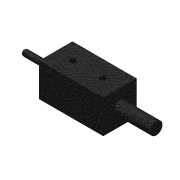
# Autodesk Inventor part: 00_JF-0530B-solenoid
Saved by Autodesk Inventor 2019.4 (Build 234330000, 330)
## iProperties
Created: 2020-11-20
Part Number: 00_JF-0530B-solenoid
Material: Generic
Document SubType Name: Modeling
Designer: diederichbenedict
Density: 1 g/cm^3
Appearance: Black Cast
Author: diederichbenedict
Autodesk Inventor part; units mm, degrees
ref_plane "YZ Plane" through (0, 0, 0) normal (1, 0, 0) x (0, 1, 0)
ref_plane "XZ Plane" through (0, 0, 0) normal (0, 1, 0) x (-1, 0, 0)
ref_plane "XY Plane" through (0, 0, 0) normal (0, 0, 1) x (1, 0, 0)
sketch "Sketch1" plane through (0, 0, 0) normal (0, 0, 1) x (1, 0, 0)
  line L0 (0, 0) -> (30, 0)
  line L1 (30, 0) -> (30, 15.6)
  line L2 (30, 15.6) -> (0, 15.6)
  line L3 (0, 15.6) -> (0, 0)
  dimension "d0" = 30
  dimension "d1" = 15.6
  constraints: 8 end point, 2 parallel, 1 horizontal, 1 perpendicular
  measures "d0" distance of L2.end L1.end
  measures "d1" distance of L1.end L0.end
extrude "Extrusion1" add sketch "Sketch1" along normal blind 15.6
sketch "Sketch2" plane through (30, 0, 0) normal (1, 0, 0) x (0, 0, -1)
  line L0 (0, 0) -> (0, 15.6) projected
  line L1 (0, 15.6) -> (-15.6, 15.6) projected
  line L2 (-15.6, 0) -> (-15.6, 15.6) projected
  line L3 (0, 0) -> (-15.6, 0) projected
  circle A0 centre (-7.8, 7.8) radius 2.9
  dimension "d4" = 5.8
  constraints: 1 centre point
  measures "d4" diameter of A0
extrude "Extrusion2" add sketch "Sketch2" along normal blind 17 contours A0
sketch "Sketch3" plane through (0, 0, 0) normal (-1, 0, 0) x (0, 0, 1)
  circle A0 centre (7.8, 7.8) radius 2.9 projected
  circle A1 centre (7.8, 7.8) radius 1.425
  point P0 (0, 0)
  dimension "d7" = 2.85
  constraints: 1 centre point, 1 coincident
  measures "d7" diameter of A1
extrude "Extrusion3" add sketch "Sketch3" along normal blind 15 contours A1
fillet "Fillet1" radius 1 1 edges at (-15, 7.8, 6.375)
sketch "Sketch4" plane through (0, 15.6, 0) normal (0, 1, 0) x (1, 0, 0)
  circle A0 centre (8, -7.8101) radius 1.4
  circle A1 centre (22, -7.8101) radius 1.4
  line L0 (30, 0) -> (30, -15.6) projected
  line L1 (0, 0) -> (0, -15.6) projected
  dimension "d11" = 2.8
  dimension "d12" = 2.8
  dimension "d13" = 8
  dimension "d14" = 8
  constraints: 2 centre point
  measures "d11" diameter of A0
  measures "d12" diameter of A1
  measures "d13" distance from line of A1.centre L0
  measures "d14" distance from line of A0.centre L1
extrude "Extrusion4" cut sketch "Sketch4" against normal blind 5
body "Solid1"
